Autodesk Inventor part; units mm, degrees
(part 10 of 13)
  spline S1362 degree 3 poles (18.9643, 15.7078) (18.9643, 15.461) (19.1644, 15.2608) (19.4112, 15.2608) knots 0 0 0 0 1 1 1 1
  line L4312 (18.9643, 15.7078) -> (18.9643, 15.461) construction
  line L4313 (18.9643, 15.461) -> (19.1644, 15.2608) construction
  line L4314 (19.1644, 15.2608) -> (19.4112, 15.2608) construction
  spline S1363 degree 3 poles (19.4112, 15.2608) (19.658, 15.2608) (19.8582, 15.461) (19.8582, 15.7078) knots 0 0 0 0 1 1 1 1
  line L4315 (19.4112, 15.2608) -> (19.658, 15.2608) construction
  line L4316 (19.658, 15.2608) -> (19.8582, 15.461) construction
  line L4317 (19.8582, 15.461) -> (19.8582, 15.7078) construction
  spline S1364 degree 3 poles (19.8582, 18.2619) (19.8582, 18.5087) (19.658, 18.7088) (19.4112, 18.7088) knots 0 0 0 0 1 1 1 1
  line L4318 (19.8582, 18.2619) -> (19.8582, 18.5087) construction
  line L4319 (19.8582, 18.5087) -> (19.658, 18.7088) construction
  line L4320 (19.658, 18.7088) -> (19.4112, 18.7088) construction
  spline S1365 degree 3 poles (19.4112, 18.7088) (19.1644, 18.7088) (18.9643, 18.5087) (18.9643, 18.2619) knots 0 0 0 0 1 1 1 1
  line L4321 (19.4112, 18.7088) -> (19.1644, 18.7088) construction
  line L4322 (19.1644, 18.7088) -> (18.9643, 18.5087) construction
  line L4323 (18.9643, 18.5087) -> (18.9643, 18.2619) construction
  spline S1366 degree 3 poles (18.9643, 18.2619) (18.9643, 18.0151) (19.1644, 17.8149) (19.4112, 17.8149) knots 0 0 0 0 1 1 1 1
  line L4324 (18.9643, 18.2619) -> (18.9643, 18.0151) construction
  line L4325 (18.9643, 18.0151) -> (19.1644, 17.8149) construction
  line L4326 (19.1644, 17.8149) -> (19.4112, 17.8149) construction
  spline S1367 degree 3 poles (19.4112, 17.8149) (19.658, 17.8149) (19.8582, 18.0151) (19.8582, 18.2619) knots 0 0 0 0 1 1 1 1
  line L4327 (19.4112, 17.8149) -> (19.658, 17.8149) construction
  line L4328 (19.658, 17.8149) -> (19.8582, 18.0151) construction
  line L4329 (19.8582, 18.0151) -> (19.8582, 18.2619) construction
  spline S1368 degree 3 poles (19.8582, 20.816) (19.8582, 21.0628) (19.658, 21.2629) (19.4112, 21.2629) knots 0 0 0 0 1 1 1 1
  line L4330 (19.8582, 20.816) -> (19.8582, 21.0628) construction
  line L4331 (19.8582, 21.0628) -> (19.658, 21.2629) construction
  line L4332 (19.658, 21.2629) -> (19.4112, 21.2629) construction
  spline S1369 degree 3 poles (19.4112, 21.2629) (19.1644, 21.2629) (18.9643, 21.0628) (18.9643, 20.816) knots 0 0 0 0 1 1 1 1
  line L4333 (19.4112, 21.2629) -> (19.1644, 21.2629) construction
  line L4334 (19.1644, 21.2629) -> (18.9643, 21.0628) construction
  line L4335 (18.9643, 21.0628) -> (18.9643, 20.816) construction
  spline S1370 degree 3 poles (18.9643, 20.816) (18.9643, 20.5692) (19.1644, 20.369) (19.4112, 20.369) knots 0 0 0 0 1 1 1 1
  line L4336 (18.9643, 20.816) -> (18.9643, 20.5692) construction
  line L4337 (18.9643, 20.5692) -> (19.1644, 20.369) construction
  line L4338 (19.1644, 20.369) -> (19.4112, 20.369) construction
  spline S1371 degree 3 poles (19.4112, 20.369) (19.658, 20.369) (19.8582, 20.5692) (19.8582, 20.816) knots 0 0 0 0 1 1 1 1
  line L4339 (19.4112, 20.369) -> (19.658, 20.369) construction
  line L4340 (19.658, 20.369) -> (19.8582, 20.5692) construction
  line L4341 (19.8582, 20.5692) -> (19.8582, 20.816) construction
  spline S1372 degree 3 poles (9.6418, 33.5866) (9.6418, 33.8334) (9.4415, 34.0334) (9.1948, 34.0334) knots 0 0 0 0 1 1 1 1
  line L4342 (9.6418, 33.5866) -> (9.6418, 33.8334) construction
  line L4343 (9.6418, 33.8334) -> (9.4415, 34.0334) construction
  line L4344 (9.4415, 34.0334) -> (9.1948, 34.0334) construction
  spline S1373 degree 3 poles (9.1948, 34.0334) (8.948, 34.0334) (8.7479, 33.8334) (8.7479, 33.5866) knots 0 0 0 0 1 1 1 1
  line L4345 (9.1948, 34.0334) -> (8.948, 34.0334) construction
  line L4346 (8.948, 34.0334) -> (8.7479, 33.8334) construction
  line L4347 (8.7479, 33.8334) -> (8.7479, 33.5866) construction
  spline S1374 degree 3 poles (8.7479, 33.5866) (8.7479, 33.3398) (8.948, 33.1395) (9.1948, 33.1395) knots 0 0 0 0 1 1 1 1
  line L4348 (8.7479, 33.5866) -> (8.7479, 33.3398) construction
  line L4349 (8.7479, 33.3398) -> (8.948, 33.1395) construction
  line L4350 (8.948, 33.1395) -> (9.1948, 33.1395) construction
  spline S1375 degree 3 poles (9.1948, 33.1395) (9.4415, 33.1395) (9.6418, 33.3398) (9.6418, 33.5866) knots 0 0 0 0 1 1 1 1
  line L4351 (9.1948, 33.1395) -> (9.4415, 33.1395) construction
  line L4352 (9.4415, 33.1395) -> (9.6418, 33.3398) construction
  line L4353 (9.6418, 33.3398) -> (9.6418, 33.5866) construction
  spline S1376 degree 3 poles (12.1959, 33.5866) (12.1959, 33.8334) (11.9957, 34.0334) (11.7489, 34.0334) knots 0 0 0 0 1 1 1 1
  line L4354 (12.1959, 33.5866) -> (12.1959, 33.8334) construction
  line L4355 (12.1959, 33.8334) -> (11.9957, 34.0334) construction
  line L4356 (11.9957, 34.0334) -> (11.7489, 34.0334) construction
  spline S1377 degree 3 poles (11.7489, 34.0334) (11.5021, 34.0334) (11.302, 33.8334) (11.302, 33.5866) knots 0 0 0 0 1 1 1 1
  line L4357 (11.7489, 34.0334) -> (11.5021, 34.0334) construction
  line L4358 (11.5021, 34.0334) -> (11.302, 33.8334) construction
  line L4359 (11.302, 33.8334) -> (11.302, 33.5866) construction
  spline S1378 degree 3 poles (11.302, 33.5866) (11.302, 33.3398) (11.5021, 33.1395) (11.7489, 33.1395) knots 0 0 0 0 1 1 1 1
  line L4360 (11.302, 33.5866) -> (11.302, 33.3398) construction
  line L4361 (11.302, 33.3398) -> (11.5021, 33.1395) construction
  line L4362 (11.5021, 33.1395) -> (11.7489, 33.1395) construction
  spline S1379 degree 3 poles (11.7489, 33.1395) (11.9957, 33.1395) (12.1959, 33.3398) (12.1959, 33.5866) knots 0 0 0 0 1 1 1 1
  line L4363 (11.7489, 33.1395) -> (11.9957, 33.1395) construction
  line L4364 (11.9957, 33.1395) -> (12.1959, 33.3398) construction
  line L4365 (12.1959, 33.3398) -> (12.1959, 33.5866) construction
  spline S1380 degree 3 poles (14.75, 33.5866) (14.75, 33.8334) (14.5498, 34.0334) (14.303, 34.0334) knots 0 0 0 0 1 1 1 1
  line L4366 (14.75, 33.5866) -> (14.75, 33.8334) construction
  line L4367 (14.75, 33.8334) -> (14.5498, 34.0334) construction
  line L4368 (14.5498, 34.0334) -> (14.303, 34.0334) construction
  spline S1381 degree 3 poles (14.303, 34.0334) (14.0562, 34.0334) (13.8561, 33.8334) (13.8561, 33.5866) knots 0 0 0 0 1 1 1 1
  line L4369 (14.303, 34.0334) -> (14.0562, 34.0334) construction
  line L4370 (14.0562, 34.0334) -> (13.8561, 33.8334) construction
  line L4371 (13.8561, 33.8334) -> (13.8561, 33.5866) construction
  spline S1382 degree 3 poles (13.8561, 33.5866) (13.8561, 33.3398) (14.0562, 33.1395) (14.303, 33.1395) knots 0 0 0 0 1 1 1 1
  line L4372 (13.8561, 33.5866) -> (13.8561, 33.3398) construction
  line L4373 (13.8561, 33.3398) -> (14.0562, 33.1395) construction
  line L4374 (14.0562, 33.1395) -> (14.303, 33.1395) construction
  spline S1383 degree 3 poles (14.303, 33.1395) (14.5498, 33.1395) (14.75, 33.3398) (14.75, 33.5866) knots 0 0 0 0 1 1 1 1
  line L4375 (14.303, 33.1395) -> (14.5498, 33.1395) construction
  line L4376 (14.5498, 33.1395) -> (14.75, 33.3398) construction
  line L4377 (14.75, 33.3398) -> (14.75, 33.5866) construction
  spline S1384 degree 3 poles (17.3041, 23.3701) (17.3041, 23.6169) (17.1039, 23.817) (16.8571, 23.817) knots 0 0 0 0 1 1 1 1
  line L4378 (17.3041, 23.3701) -> (17.3041, 23.6169) construction
  line L4379 (17.3041, 23.6169) -> (17.1039, 23.817) construction
  line L4380 (17.1039, 23.817) -> (16.8571, 23.817) construction
  spline S1385 degree 3 poles (16.8571, 23.817) (16.6103, 23.817) (16.4102, 23.6169) (16.4102, 23.3701) knots 0 0 0 0 1 1 1 1
  line L4381 (16.8571, 23.817) -> (16.6103, 23.817) construction
  line L4382 (16.6103, 23.817) -> (16.4102, 23.6169) construction
  line L4383 (16.4102, 23.6169) -> (16.4102, 23.3701) construction
  spline S1386 degree 3 poles (16.4102, 23.3701) (16.4102, 23.1233) (16.6103, 22.9231) (16.8571, 22.9231) knots 0 0 0 0 1 1 1 1
  line L4384 (16.4102, 23.3701) -> (16.4102, 23.1233) construction
  line L4385 (16.4102, 23.1233) -> (16.6103, 22.9231) construction
  line L4386 (16.6103, 22.9231) -> (16.8571, 22.9231) construction
  spline S1387 degree 3 poles (16.8571, 22.9231) (17.1039, 22.9231) (17.3041, 23.1233) (17.3041, 23.3701) knots 0 0 0 0 1 1 1 1
  line L4387 (16.8571, 22.9231) -> (17.1039, 22.9231) construction
  line L4388 (17.1039, 22.9231) -> (17.3041, 23.1233) construction
  line L4389 (17.3041, 23.1233) -> (17.3041, 23.3701) construction
  spline S1388 degree 3 poles (22.7955, 22.2718) (22.7955, 22.5186) (22.5952, 22.7188) (22.3485, 22.7188) knots 0 0 0 0 1 1 1 1
  line L4390 (22.7955, 22.2718) -> (22.7955, 22.5186) construction
  line L4391 (22.7955, 22.5186) -> (22.5952, 22.7188) construction
  line L4392 (22.5952, 22.7188) -> (22.3485, 22.7188) construction
  spline S1389 degree 3 poles (22.3485, 22.7188) (22.1017, 22.7188) (21.9014, 22.5186) (21.9014, 22.2718) knots 0 0 0 0 1 1 1 1
  line L4393 (22.3485, 22.7188) -> (22.1017, 22.7188) construction
  line L4394 (22.1017, 22.7188) -> (21.9014, 22.5186) construction
  line L4395 (21.9014, 22.5186) -> (21.9014, 22.2718) construction
  spline S1390 degree 3 poles (21.9014, 22.2718) (21.9014, 22.025) (22.1017, 21.8248) (22.3485, 21.8248) knots 0 0 0 0 1 1 1 1
  line L4396 (21.9014, 22.2718) -> (21.9014, 22.025) construction
  line L4397 (21.9014, 22.025) -> (22.1017, 21.8248) construction
  line L4398 (22.1017, 21.8248) -> (22.3485, 21.8248) construction
  spline S1391 degree 3 poles (22.3485, 21.8248) (22.5952, 21.8248) (22.7955, 22.025) (22.7955, 22.2718) knots 0 0 0 0 1 1 1 1
  line L4399 (22.3485, 21.8248) -> (22.5952, 21.8248) construction
  line L4400 (22.5952, 21.8248) -> (22.7955, 22.025) construction
  line L4401 (22.7955, 22.025) -> (22.7955, 22.2718) construction
  spline S1392 degree 3 poles (25.3496, 22.2718) (25.3496, 22.5186) (25.1494, 22.7188) (24.9026, 22.7188) knots 0 0 0 0 1 1 1 1
  line L4402 (25.3496, 22.2718) -> (25.3496, 22.5186) construction
  line L4403 (25.3496, 22.5186) -> (25.1494, 22.7188) construction
  line L4404 (25.1494, 22.7188) -> (24.9026, 22.7188) construction
  spline S1393 degree 3 poles (24.9026, 22.7188) (24.6558, 22.7188) (24.4555, 22.5186) (24.4555, 22.2718) knots 0 0 0 0 1 1 1 1
  line L4405 (24.9026, 22.7188) -> (24.6558, 22.7188) construction
  line L4406 (24.6558, 22.7188) -> (24.4555, 22.5186) construction
  line L4407 (24.4555, 22.5186) -> (24.4555, 22.2718) construction
  spline S1394 degree 3 poles (24.4555, 22.2718) (24.4555, 22.025) (24.6558, 21.8248) (24.9026, 21.8248) knots 0 0 0 0 1 1 1 1
  line L4408 (24.4555, 22.2718) -> (24.4555, 22.025) construction
  line L4409 (24.4555, 22.025) -> (24.6558, 21.8248) construction
  line L4410 (24.6558, 21.8248) -> (24.9026, 21.8248) construction
  spline S1395 degree 3 poles (24.9026, 21.8248) (25.1494, 21.8248) (25.3496, 22.025) (25.3496, 22.2718) knots 0 0 0 0 1 1 1 1
  line L4411 (24.9026, 21.8248) -> (25.1494, 21.8248) construction
  line L4412 (25.1494, 21.8248) -> (25.3496, 22.025) construction
  line L4413 (25.3496, 22.025) -> (25.3496, 22.2718) construction
  spline S1396 degree 3 poles (22.7955, 24.8259) (22.7955, 25.0727) (22.5952, 25.2729) (22.3485, 25.2729) knots 0 0 0 0 1 1 1 1
  line L4414 (22.7955, 24.8259) -> (22.7955, 25.0727) construction
  line L4415 (22.7955, 25.0727) -> (22.5952, 25.2729) construction
  line L4416 (22.5952, 25.2729) -> (22.3485, 25.2729) construction
  spline S1397 degree 3 poles (22.3485, 25.2729) (22.1017, 25.2729) (21.9014, 25.0727) (21.9014, 24.8259) knots 0 0 0 0 1 1 1 1
  line L4417 (22.3485, 25.2729) -> (22.1017, 25.2729) construction
  line L4418 (22.1017, 25.2729) -> (21.9014, 25.0727) construction
  line L4419 (21.9014, 25.0727) -> (21.9014, 24.8259) construction
  spline S1398 degree 3 poles (21.9014, 24.8259) (21.9014, 24.5792) (22.1017, 24.3789) (22.3485, 24.3789) knots 0 0 0 0 1 1 1 1
  line L4420 (21.9014, 24.8259) -> (21.9014, 24.5792) construction
  line L4421 (21.9014, 24.5792) -> (22.1017, 24.3789) construction
  line L4422 (22.1017, 24.3789) -> (22.3485, 24.3789) construction
  spline S1399 degree 3 poles (22.3485, 24.3789) (22.5952, 24.3789) (22.7955, 24.5792) (22.7955, 24.8259) knots 0 0 0 0 1 1 1 1
  line L4423 (22.3485, 24.3789) -> (22.5952, 24.3789) construction
  line L4424 (22.5952, 24.3789) -> (22.7955, 24.5792) construction
  line L4425 (22.7955, 24.5792) -> (22.7955, 24.8259) construction
  spline S1400 degree 3 poles (25.3496, 24.8259) (25.3496, 25.0727) (25.1494, 25.2729) (24.9026, 25.2729) knots 0 0 0 0 1 1 1 1
  line L4426 (25.3496, 24.8259) -> (25.3496, 25.0727) construction
  line L4427 (25.3496, 25.0727) -> (25.1494, 25.2729) construction
  line L4428 (25.1494, 25.2729) -> (24.9026, 25.2729) construction
  spline S1401 degree 3 poles (24.9026, 25.2729) (24.6558, 25.2729) (24.4555, 25.0727) (24.4555, 24.8259) knots 0 0 0 0 1 1 1 1
  line L4429 (24.9026, 25.2729) -> (24.6558, 25.2729) construction
  line L4430 (24.6558, 25.2729) -> (24.4555, 25.0727) construction
  line L4431 (24.4555, 25.0727) -> (24.4555, 24.8259) construction
  spline S1402 degree 3 poles (24.4555, 24.8259) (24.4555, 24.5792) (24.6558, 24.3789) (24.9026, 24.3789) knots 0 0 0 0 1 1 1 1
  line L4432 (24.4555, 24.8259) -> (24.4555, 24.5792) construction
  line L4433 (24.4555, 24.5792) -> (24.6558, 24.3789) construction
  line L4434 (24.6558, 24.3789) -> (24.9026, 24.3789) construction
  spline S1403 degree 3 poles (24.9026, 24.3789) (25.1494, 24.3789) (25.3496, 24.5792) (25.3496, 24.8259) knots 0 0 0 0 1 1 1 1
  line L4435 (24.9026, 24.3789) -> (25.1494, 24.3789) construction
  line L4436 (25.1494, 24.3789) -> (25.3496, 24.5792) construction
  line L4437 (25.3496, 24.5792) -> (25.3496, 24.8259) construction
  spline S1404 degree 3 poles (19.8582, 23.3701) (19.8582, 23.6169) (19.658, 23.817) (19.4112, 23.817) knots 0 0 0 0 1 1 1 1
  line L4438 (19.8582, 23.3701) -> (19.8582, 23.6169) construction
  line L4439 (19.8582, 23.6169) -> (19.658, 23.817) construction
  line L4440 (19.658, 23.817) -> (19.4112, 23.817) construction
  spline S1405 degree 3 poles (19.4112, 23.817) (19.1644, 23.817) (18.9643, 23.6169) (18.9643, 23.3701) knots 0 0 0 0 1 1 1 1
  line L4441 (19.4112, 23.817) -> (19.1644, 23.817) construction
  line L4442 (19.1644, 23.817) -> (18.9643, 23.6169) construction
  line L4443 (18.9643, 23.6169) -> (18.9643, 23.3701) construction
  spline S1406 degree 3 poles (18.9643, 23.3701) (18.9643, 23.1233) (19.1644, 22.9231) (19.4112, 22.9231) knots 0 0 0 0 1 1 1 1
  line L4444 (18.9643, 23.3701) -> (18.9643, 23.1233) construction
  line L4445 (18.9643, 23.1233) -> (19.1644, 22.9231) construction
  line L4446 (19.1644, 22.9231) -> (19.4112, 22.9231) construction
  spline S1407 degree 3 poles (19.4112, 22.9231) (19.658, 22.9231) (19.8582, 23.1233) (19.8582, 23.3701) knots 0 0 0 0 1 1 1 1
  line L4447 (19.4112, 22.9231) -> (19.658, 22.9231) construction
  line L4448 (19.658, 22.9231) -> (19.8582, 23.1233) construction
  line L4449 (19.8582, 23.1233) -> (19.8582, 23.3701) construction
  spline S1408 degree 3 poles (19.8582, 25.9242) (19.8582, 26.171) (19.658, 26.3711) (19.4112, 26.3711) knots 0 0 0 0 1 1 1 1
  line L4450 (19.8582, 25.9242) -> (19.8582, 26.171) construction
  line L4451 (19.8582, 26.171) -> (19.658, 26.3711) construction
  line L4452 (19.658, 26.3711) -> (19.4112, 26.3711) construction
  spline S1409 degree 3 poles (19.4112, 26.3711) (19.1644, 26.3711) (18.9643, 26.171) (18.9643, 25.9242) knots 0 0 0 0 1 1 1 1
  line L4453 (19.4112, 26.3711) -> (19.1644, 26.3711) construction
  line L4454 (19.1644, 26.3711) -> (18.9643, 26.171) construction
  line L4455 (18.9643, 26.171) -> (18.9643, 25.9242) construction
  spline S1410 degree 3 poles (18.9643, 25.9242) (18.9643, 25.6775) (19.1644, 25.4772) (19.4112, 25.4772) knots 0 0 0 0 1 1 1 1
  line L4456 (18.9643, 25.9242) -> (18.9643, 25.6775) construction
  line L4457 (18.9643, 25.6775) -> (19.1644, 25.4772) construction
  line L4458 (19.1644, 25.4772) -> (19.4112, 25.4772) construction
  spline S1411 degree 3 poles (19.4112, 25.4772) (19.658, 25.4772) (19.8582, 25.6775) (19.8582, 25.9242) knots 0 0 0 0 1 1 1 1
  line L4459 (19.4112, 25.4772) -> (19.658, 25.4772) construction
  line L4460 (19.658, 25.4772) -> (19.8582, 25.6775) construction
  line L4461 (19.8582, 25.6775) -> (19.8582, 25.9242) construction
  spline S1412 degree 3 poles (19.8582, 28.4784) (19.8582, 28.7251) (19.658, 28.9252) (19.4112, 28.9252) knots 0 0 0 0 1 1 1 1
  line L4462 (19.8582, 28.4784) -> (19.8582, 28.7251) construction
  line L4463 (19.8582, 28.7251) -> (19.658, 28.9252) construction
  line L4464 (19.658, 28.9252) -> (19.4112, 28.9252) construction
  spline S1413 degree 3 poles (19.4112, 28.9252) (19.1644, 28.9252) (18.9643, 28.7251) (18.9643, 28.4784) knots 0 0 0 0 1 1 1 1
  line L4465 (19.4112, 28.9252) -> (19.1644, 28.9252) construction
  line L4466 (19.1644, 28.9252) -> (18.9643, 28.7251) construction
  line L4467 (18.9643, 28.7251) -> (18.9643, 28.4784) construction
  spline S1414 degree 3 poles (18.9643, 28.4784) (18.9643, 28.2316) (19.1644, 28.0313) (19.4112, 28.0313) knots 0 0 0 0 1 1 1 1
  line L4468 (18.9643, 28.4784) -> (18.9643, 28.2316) construction
  line L4469 (18.9643, 28.2316) -> (19.1644, 28.0313) construction
  line L4470 (19.1644, 28.0313) -> (19.4112, 28.0313) construction
  spline S1415 degree 3 poles (19.4112, 28.0313) (19.658, 28.0313) (19.8582, 28.2316) (19.8582, 28.4784) knots 0 0 0 0 1 1 1 1
  line L4471 (19.4112, 28.0313) -> (19.658, 28.0313) construction
  line L4472 (19.658, 28.0313) -> (19.8582, 28.2316) construction
  line L4473 (19.8582, 28.2316) -> (19.8582, 28.4784) construction
  spline S1416 degree 3 poles (19.8582, 31.0325) (19.8582, 31.2793) (19.658, 31.4793) (19.4112, 31.4793) knots 0 0 0 0 1 1 1 1
  line L4474 (19.8582, 31.0325) -> (19.8582, 31.2793) construction
  line L4475 (19.8582, 31.2793) -> (19.658, 31.4793) construction
  line L4476 (19.658, 31.4793) -> (19.4112, 31.4793) construction
  spline S1417 degree 3 poles (19.4112, 31.4793) (19.1644, 31.4793) (18.9643, 31.2793) (18.9643, 31.0325) knots 0 0 0 0 1 1 1 1
  line L4477 (19.4112, 31.4793) -> (19.1644, 31.4793) construction
  line L4478 (19.1644, 31.4793) -> (18.9643, 31.2793) construction
  line L4479 (18.9643, 31.2793) -> (18.9643, 31.0325) construction
  spline S1418 degree 3 poles (18.9643, 31.0325) (18.9643, 30.7857) (19.1644, 30.5854) (19.4112, 30.5854) knots 0 0 0 0 1 1 1 1
  line L4480 (18.9643, 31.0325) -> (18.9643, 30.7857) construction
  line L4481 (18.9643, 30.7857) -> (19.1644, 30.5854) construction
  line L4482 (19.1644, 30.5854) -> (19.4112, 30.5854) construction
  spline S1419 degree 3 poles (19.4112, 30.5854) (19.658, 30.5854) (19.8582, 30.7857) (19.8582, 31.0325) knots 0 0 0 0 1 1 1 1
  line L4483 (19.4112, 30.5854) -> (19.658, 30.5854) construction
  line L4484 (19.658, 30.5854) -> (19.8582, 30.7857) construction
  line L4485 (19.8582, 30.7857) -> (19.8582, 31.0325) construction
  spline S1420 degree 3 poles (17.3041, 25.9242) (17.3041, 26.171) (17.1039, 26.3711) (16.8571, 26.3711) knots 0 0 0 0 1 1 1 1
  line L4486 (17.3041, 25.9242) -> (17.3041, 26.171) construction
  line L4487 (17.3041, 26.171) -> (17.1039, 26.3711) construction
  line L4488 (17.1039, 26.3711) -> (16.8571, 26.3711) construction
  spline S1421 degree 3 poles (16.8571, 26.3711) (16.6103, 26.3711) (16.4102, 26.171) (16.4102, 25.9242) knots 0 0 0 0 1 1 1 1
  line L4489 (16.8571, 26.3711) -> (16.6103, 26.3711) construction
  line L4490 (16.6103, 26.3711) -> (16.4102, 26.171) construction
  line L4491 (16.4102, 26.171) -> (16.4102, 25.9242) construction
  spline S1422 degree 3 poles (16.4102, 25.9242) (16.4102, 25.6775) (16.6103, 25.4772) (16.8571, 25.4772) knots 0 0 0 0 1 1 1 1
  line L4492 (16.4102, 25.9242) -> (16.4102, 25.6775) construction
  line L4493 (16.4102, 25.6775) -> (16.6103, 25.4772) construction
  line L4494 (16.6103, 25.4772) -> (16.8571, 25.4772) construction
  spline S1423 degree 3 poles (16.8571, 25.4772) (17.1039, 25.4772) (17.3041, 25.6775) (17.3041, 25.9242) knots 0 0 0 0 1 1 1 1
  line L4495 (16.8571, 25.4772) -> (17.1039, 25.4772) construction
  line L4496 (17.1039, 25.4772) -> (17.3041, 25.6775) construction
  line L4497 (17.3041, 25.6775) -> (17.3041, 25.9242) construction
  spline S1424 degree 3 poles (17.3041, 28.4784) (17.3041, 28.7251) (17.1039, 28.9252) (16.8571, 28.9252) knots 0 0 0 0 1 1 1 1
  line L4498 (17.3041, 28.4784) -> (17.3041, 28.7251) construction
  line L4499 (17.3041, 28.7251) -> (17.1039, 28.9252) construction
  line L4500 (17.1039, 28.9252) -> (16.8571, 28.9252) construction
  spline S1425 degree 3 poles (16.8571, 28.9252) (16.6103, 28.9252) (16.4102, 28.7251) (16.4102, 28.4784) knots 0 0 0 0 1 1 1 1
  line L4501 (16.8571, 28.9252) -> (16.6103, 28.9252) construction
  line L4502 (16.6103, 28.9252) -> (16.4102, 28.7251) construction
  line L4503 (16.4102, 28.7251) -> (16.4102, 28.4784) construction
  spline S1426 degree 3 poles (16.4102, 28.4784) (16.4102, 28.2316) (16.6103, 28.0313) (16.8571, 28.0313) knots 0 0 0 0 1 1 1 1
  line L4504 (16.4102, 28.4784) -> (16.4102, 28.2316) construction
  line L4505 (16.4102, 28.2316) -> (16.6103, 28.0313) construction
  line L4506 (16.6103, 28.0313) -> (16.8571, 28.0313) construction
  spline S1427 degree 3 poles (16.8571, 28.0313) (17.1039, 28.0313) (17.3041, 28.2316) (17.3041, 28.4784) knots 0 0 0 0 1 1 1 1
  line L4507 (16.8571, 28.0313) -> (17.1039, 28.0313) construction
  line L4508 (17.1039, 28.0313) -> (17.3041, 28.2316) construction
  line L4509 (17.3041, 28.2316) -> (17.3041, 28.4784) construction
  spline S1428 degree 3 poles (17.3041, 31.0325) (17.3041, 31.2793) (17.1039, 31.4793) (16.8571, 31.4793) knots 0 0 0 0 1 1 1 1
  line L4510 (17.3041, 31.0325) -> (17.3041, 31.2793) construction
  line L4511 (17.3041, 31.2793) -> (17.1039, 31.4793) construction
  line L4512 (17.1039, 31.4793) -> (16.8571, 31.4793) construction
  spline S1429 degree 3 poles (16.8571, 31.4793) (16.6103, 31.4793) (16.4102, 31.2793) (16.4102, 31.0325) knots 0 0 0 0 1 1 1 1
  line L4513 (16.8571, 31.4793) -> (16.6103, 31.4793) construction
  line L4514 (16.6103, 31.4793) -> (16.4102, 31.2793) construction
  line L4515 (16.4102, 31.2793) -> (16.4102, 31.0325) construction
  spline S1430 degree 3 poles (16.4102, 31.0325) (16.4102, 30.7857) (16.6103, 30.5854) (16.8571, 30.5854) knots 0 0 0 0 1 1 1 1
  line L4516 (16.4102, 31.0325) -> (16.4102, 30.7857) construction
  line L4517 (16.4102, 30.7857) -> (16.6103, 30.5854) construction
  line L4518 (16.6103, 30.5854) -> (16.8571, 30.5854) construction
  spline S1431 degree 3 poles (16.8571, 30.5854) (17.1039, 30.5854) (17.3041, 30.7857) (17.3041, 31.0325) knots 0 0 0 0 1 1 1 1
  line L4519 (16.8571, 30.5854) -> (17.1039, 30.5854) construction
  line L4520 (17.1039, 30.5854) -> (17.3041, 30.7857) construction
  line L4521 (17.3041, 30.7857) -> (17.3041, 31.0325) construction
  spline S1432 degree 3 poles (37.737, 33.5866) (37.737, 33.8334) (37.5369, 34.0334) (37.29, 34.0334) knots 0 0 0 0 1 1 1 1
  line L4522 (37.737, 33.5866) -> (37.737, 33.8334) construction
  line L4523 (37.737, 33.8334) -> (37.5369, 34.0334) construction
  line L4524 (37.5369, 34.0334) -> (37.29, 34.0334) construction
  spline S1433 degree 3 poles (37.29, 34.0334) (37.0431, 34.0334) (36.843, 33.8334) (36.843, 33.5866) knots 0 0 0 0 1 1 1 1
  line L4525 (37.29, 34.0334) -> (37.0431, 34.0334) construction
  line L4526 (37.0431, 34.0334) -> (36.843, 33.8334) construction
  line L4527 (36.843, 33.8334) -> (36.843, 33.5866) construction
  spline S1434 degree 3 poles (36.843, 33.5866) (36.843, 33.3398) (37.0431, 33.1395) (37.29, 33.1395) knots 0 0 0 0 1 1 1 1
  line L4528 (36.843, 33.5866) -> (36.843, 33.3398) construction
  line L4529 (36.843, 33.3398) -> (37.0431, 33.1395) construction
  line L4530 (37.0431, 33.1395) -> (37.29, 33.1395) construction
  spline S1435 degree 3 poles (37.29, 33.1395) (37.5369, 33.1395) (37.737, 33.3398) (37.737, 33.5866) knots 0 0 0 0 1 1 1 1
  line L4531 (37.29, 33.1395) -> (37.5369, 33.1395) construction
  line L4532 (37.5369, 33.1395) -> (37.737, 33.3398) construction
  line L4533 (37.737, 33.3398) -> (37.737, 33.5866) construction
  spline S1436 degree 3 poles (40.2911, 33.5866) (40.2911, 33.8334) (40.091, 34.0334) (39.8441, 34.0334) knots 0 0 0 0 1 1 1 1
  line L4534 (40.2911, 33.5866) -> (40.2911, 33.8334) construction
  line L4535 (40.2911, 33.8334) -> (40.091, 34.0334) construction
  line L4536 (40.091, 34.0334) -> (39.8441, 34.0334) construction
  spline S1437 degree 3 poles (39.8441, 34.0334) (39.5972, 34.0334) (39.3971, 33.8334) (39.3971, 33.5866) knots 0 0 0 0 1 1 1 1
  line L4537 (39.8441, 34.0334) -> (39.5972, 34.0334) construction
  line L4538 (39.5972, 34.0334) -> (39.3971, 33.8334) construction
  line L4539 (39.3971, 33.8334) -> (39.3971, 33.5866) construction
  spline S1438 degree 3 poles (39.3971, 33.5866) (39.3971, 33.3398) (39.5972, 33.1395) (39.8441, 33.1395) knots 0 0 0 0 1 1 1 1
  line L4540 (39.3971, 33.5866) -> (39.3971, 33.3398) construction
  line L4541 (39.3971, 33.3398) -> (39.5972, 33.1395) construction
  line L4542 (39.5972, 33.1395) -> (39.8441, 33.1395) construction
  spline S1439 degree 3 poles (39.8441, 33.1395) (40.091, 33.1395) (40.2911, 33.3398) (40.2911, 33.5866) knots 0 0 0 0 1 1 1 1
  line L4543 (39.8441, 33.1395) -> (40.091, 33.1395) construction
  line L4544 (40.091, 33.1395) -> (40.2911, 33.3398) construction
  line L4545 (40.2911, 33.3398) -> (40.2911, 33.5866) construction
  spline S1440 degree 3 poles (42.8452, 33.5866) (42.8452, 33.8334) (42.6451, 34.0334) (42.3982, 34.0334) knots 0 0 0 0 1 1 1 1
  line L4546 (42.8452, 33.5866) -> (42.8452, 33.8334) construction
  line L4547 (42.8452, 33.8334) -> (42.6451, 34.0334) construction
  line L4548 (42.6451, 34.0334) -> (42.3982, 34.0334) construction
  spline S1441 degree 3 poles (42.3982, 34.0334) (42.1513, 34.0334) (41.9512, 33.8334) (41.9512, 33.5866) knots 0 0 0 0 1 1 1 1
  line L4549 (42.3982, 34.0334) -> (42.1513, 34.0334) construction
  line L4550 (42.1513, 34.0334) -> (41.9512, 33.8334) construction
  line L4551 (41.9512, 33.8334) -> (41.9512, 33.5866) construction
  spline S1442 degree 3 poles (41.9512, 33.5866) (41.9512, 33.3398) (42.1513, 33.1395) (42.3982, 33.1395) knots 0 0 0 0 1 1 1 1
  line L4552 (41.9512, 33.5866) -> (41.9512, 33.3398) construction
  line L4553 (41.9512, 33.3398) -> (42.1513, 33.1395) construction
  line L4554 (42.1513, 33.1395) -> (42.3982, 33.1395) construction
  spline S1443 degree 3 poles (42.3982, 33.1395) (42.6451, 33.1395) (42.8452, 33.3398) (42.8452, 33.5866) knots 0 0 0 0 1 1 1 1
  line L4555 (42.3982, 33.1395) -> (42.6451, 33.1395) construction
  line L4556 (42.6451, 33.1395) -> (42.8452, 33.3398) construction
  line L4557 (42.8452, 33.3398) -> (42.8452, 33.5866) construction
  spline S1444 degree 3 poles (45.3993, 33.5866) (45.3993, 33.8334) (45.1992, 34.0334) (44.9523, 34.0334) knots 0 0 0 0 1 1 1 1
  line L4558 (45.3993, 33.5866) -> (45.3993, 33.8334) construction
  line L4559 (45.3993, 33.8334) -> (45.1992, 34.0334) construction
  line L4560 (45.1992, 34.0334) -> (44.9523, 34.0334) construction
  spline S1445 degree 3 poles (44.9523, 34.0334) (44.7054, 34.0334) (44.5054, 33.8334) (44.5054, 33.5866) knots 0 0 0 0 1 1 1 1
  line L4561 (44.9523, 34.0334) -> (44.7054, 34.0334) construction
  line L4562 (44.7054, 34.0334) -> (44.5054, 33.8334) construction
  line L4563 (44.5054, 33.8334) -> (44.5054, 33.5866) construction
  spline S1446 degree 3 poles (44.5054, 33.5866) (44.5054, 33.3398) (44.7054, 33.1395) (44.9523, 33.1395) knots 0 0 0 0 1 1 1 1
  line L4564 (44.5054, 33.5866) -> (44.5054, 33.3398) construction
  line L4565 (44.5054, 33.3398) -> (44.7054, 33.1395) construction
  line L4566 (44.7054, 33.1395) -> (44.9523, 33.1395) construction
  spline S1447 degree 3 poles (44.9523, 33.1395) (45.1992, 33.1395) (45.3993, 33.3398) (45.3993, 33.5866) knots 0 0 0 0 1 1 1 1
  line L4567 (44.9523, 33.1395) -> (45.1992, 33.1395) construction
  line L4568 (45.1992, 33.1395) -> (45.3993, 33.3398) construction
  line L4569 (45.3993, 33.3398) -> (45.3993, 33.5866) construction
  spline S1448 degree 3 poles (33.9058, 0.3832) (33.9058, 0.6299) (33.7056, 0.83) (33.4588, 0.83) knots 0 0 0 0 1 1 1 1
  line L4570 (33.9058, 0.3832) -> (33.9058, 0.6299) construction
  line L4571 (33.9058, 0.6299) -> (33.7056, 0.83) construction
  line L4572 (33.7056, 0.83) -> (33.4588, 0.83) construction
  spline S1449 degree 3 poles (33.4588, 0.83) (33.212, 0.83) (33.0119, 0.6299) (33.0119, 0.3832) knots 0 0 0 0 1 1 1 1
  line L4573 (33.4588, 0.83) -> (33.212, 0.83) construction
  line L4574 (33.212, 0.83) -> (33.0119, 0.6299) construction
  line L4575 (33.0119, 0.6299) -> (33.0119, 0.3832) construction
  spline S1450 degree 3 poles (33.0119, 0.3832) (33.0119, 0.1364) (33.212, -0.0639) (33.4588, -0.0639) knots 0 0 0 0 1 1 1 1
  line L4576 (33.0119, 0.3832) -> (33.0119, 0.1364) construction
  line L4577 (33.0119, 0.1364) -> (33.212, -0.0639) construction
  line L4578 (33.212, -0.0639) -> (33.4588, -0.0639) construction
  spline S1451 degree 3 poles (33.4588, -0.0639) (33.7056, -0.0639) (33.9058, 0.1364) (33.9058, 0.3832) knots 0 0 0 0 1 1 1 1
  line L4579 (33.4588, -0.0639) -> (33.7056, -0.0639) construction
  line L4580 (33.7056, -0.0639) -> (33.9058, 0.1364) construction
  line L4581 (33.9058, 0.1364) -> (33.9058, 0.3832) construction
  spline S1452 degree 3 poles (31.3517, 0.3832) (31.3517, 0.6299) (31.1515, 0.83) (30.9047, 0.83) knots 0 0 0 0 1 1 1 1
  line L4582 (31.3517, 0.3832) -> (31.3517, 0.6299) construction
  line L4583 (31.3517, 0.6299) -> (31.1515, 0.83) construction
  line L4584 (31.1515, 0.83) -> (30.9047, 0.83) construction
  spline S1453 degree 3 poles (30.9047, 0.83) (30.6579, 0.83) (30.4578, 0.6299) (30.4578, 0.3832) knots 0 0 0 0 1 1 1 1
  line L4585 (30.9047, 0.83) -> (30.6579, 0.83) construction
  line L4586 (30.6579, 0.83) -> (30.4578, 0.6299) construction
  line L4587 (30.4578, 0.6299) -> (30.4578, 0.3832) construction
  spline S1454 degree 3 poles (30.4578, 0.3832) (30.4578, 0.1364) (30.6579, -0.0639) (30.9047, -0.0639) knots 0 0 0 0 1 1 1 1
  line L4588 (30.4578, 0.3832) -> (30.4578, 0.1364) construction
  line L4589 (30.4578, 0.1364) -> (30.6579, -0.0639) construction
  line L4590 (30.6579, -0.0639) -> (30.9047, -0.0639) construction
  spline S1455 degree 3 poles (30.9047, -0.0639) (31.1515, -0.0639) (31.3517, 0.1364) (31.3517, 0.3832) knots 0 0 0 0 1 1 1 1
  line L4591 (30.9047, -0.0639) -> (31.1515, -0.0639) construction
  line L4592 (31.1515, -0.0639) -> (31.3517, 0.1364) construction
  line L4593 (31.3517, 0.1364) -> (31.3517, 0.3832) construction
  spline S1456 degree 3 poles (28.7976, 0.3832) (28.7976, 0.6299) (28.5974, 0.83) (28.3506, 0.83) knots 0 0 0 0 1 1 1 1
  line L4594 (28.7976, 0.3832) -> (28.7976, 0.6299) construction
  line L4595 (28.7976, 0.6299) -> (28.5974, 0.83) construction
  line L4596 (28.5974, 0.83) -> (28.3506, 0.83) construction
  spline S1457 degree 3 poles (28.3506, 0.83) (28.1038, 0.83) (27.9037, 0.6299) (27.9037, 0.3832) knots 0 0 0 0 1 1 1 1
  line L4597 (28.3506, 0.83) -> (28.1038, 0.83) construction
  line L4598 (28.1038, 0.83) -> (27.9037, 0.6299) construction
  line L4599 (27.9037, 0.6299) -> (27.9037, 0.3832) construction
  spline S1458 degree 3 poles (27.9037, 0.3832) (27.9037, 0.1364) (28.1038, -0.0639) (28.3506, -0.0639) knots 0 0 0 0 1 1 1 1
  line L4600 (27.9037, 0.3832) -> (27.9037, 0.1364) construction
  line L4601 (27.9037, 0.1364) -> (28.1038, -0.0639) construction
  line L4602 (28.1038, -0.0639) -> (28.3506, -0.0639) construction
  spline S1459 degree 3 poles (28.3506, -0.0639) (28.5974, -0.0639) (28.7976, 0.1364) (28.7976, 0.3832) knots 0 0 0 0 1 1 1 1
  line L4603 (28.3506, -0.0639) -> (28.5974, -0.0639) construction
  line L4604 (28.5974, -0.0639) -> (28.7976, 0.1364) construction
  line L4605 (28.7976, 0.1364) -> (28.7976, 0.3832) construction
  spline S1460 degree 3 poles (42.8452, 0.3832) (42.8452, 0.6299) (42.6451, 0.83) (42.3982, 0.83) knots 0 0 0 0 1 1 1 1
  line L4606 (42.8452, 0.3832) -> (42.8452, 0.6299) construction
  line L4607 (42.8452, 0.6299) -> (42.6451, 0.83) construction
  line L4608 (42.6451, 0.83) -> (42.3982, 0.83) construction
  spline S1461 degree 3 poles (42.3982, 0.83) (42.1513, 0.83) (41.9512, 0.6299) (41.9512, 0.3832) knots 0 0 0 0 1 1 1 1
  line L4609 (42.3982, 0.83) -> (42.1513, 0.83) construction
  line L4610 (42.1513, 0.83) -> (41.9512, 0.6299) construction
  line L4611 (41.9512, 0.6299) -> (41.9512, 0.3832) construction
  spline S1462 degree 3 poles (41.9512, 0.3832) (41.9512, 0.1364) (42.1513, -0.0639) (42.3982, -0.0639) knots 0 0 0 0 1 1 1 1
  line L4612 (41.9512, 0.3832) -> (41.9512, 0.1364) construction
  line L4613 (41.9512, 0.1364) -> (42.1513, -0.0639) construction
  line L4614 (42.1513, -0.0639) -> (42.3982, -0.0639) construction
  spline S1463 degree 3 poles (42.3982, -0.0639) (42.6451, -0.0639) (42.8452, 0.1364) (42.8452, 0.3832) knots 0 0 0 0 1 1 1 1
  line L4615 (42.3982, -0.0639) -> (42.6451, -0.0639) construction
  line L4616 (42.6451, -0.0639) -> (42.8452, 0.1364) construction
  line L4617 (42.8452, 0.1364) -> (42.8452, 0.3832) construction
  spline S1464 degree 3 poles (35.1829, 2.9373) (35.1829, 3.1841) (34.9826, 3.3841) (34.7358, 3.3841) knots 0 0 0 0 1 1 1 1
  line L4618 (35.1829, 2.9373) -> (35.1829, 3.1841) construction
  line L4619 (35.1829, 3.1841) -> (34.9826, 3.3841) construction
  line L4620 (34.9826, 3.3841) -> (34.7358, 3.3841) construction
  spline S1465 degree 3 poles (34.7358, 3.3841) (34.4891, 3.3841) (34.289, 3.1841) (34.289, 2.9373) knots 0 0 0 0 1 1 1 1
  line L4621 (34.7358, 3.3841) -> (34.4891, 3.3841) construction
  line L4622 (34.4891, 3.3841) -> (34.289, 3.1841) construction
  line L4623 (34.289, 3.1841) -> (34.289, 2.9373) construction
  spline S1466 degree 3 poles (34.289, 2.9373) (34.289, 2.6905) (34.4891, 2.4902) (34.7358, 2.4902) knots 0 0 0 0 1 1 1 1
  line L4624 (34.289, 2.9373) -> (34.289, 2.6905) construction
  line L4625 (34.289, 2.6905) -> (34.4891, 2.4902) construction
  line L4626 (34.4891, 2.4902) -> (34.7358, 2.4902) construction
  spline S1467 degree 3 poles (34.7358, 2.4902) (34.9826, 2.4902) (35.1829, 2.6905) (35.1829, 2.9373) knots 0 0 0 0 1 1 1 1
  line L4627 (34.7358, 2.4902) -> (34.9826, 2.4902) construction
  line L4628 (34.9826, 2.4902) -> (35.1829, 2.6905) construction
  line L4629 (35.1829, 2.6905) -> (35.1829, 2.9373) construction
  spline S1468 degree 3 poles (35.1829, 5.4914) (35.1829, 5.7382) (34.9826, 5.9382) (34.7358, 5.9382) knots 0 0 0 0 1 1 1 1
  line L4630 (35.1829, 5.4914) -> (35.1829, 5.7382) construction
  line L4631 (35.1829, 5.7382) -> (34.9826, 5.9382) construction
  line L4632 (34.9826, 5.9382) -> (34.7358, 5.9382) construction
  spline S1469 degree 3 poles (34.7358, 5.9382) (34.4891, 5.9382) (34.289, 5.7382) (34.289, 5.4914) knots 0 0 0 0 1 1 1 1
  line L4633 (34.7358, 5.9382) -> (34.4891, 5.9382) construction
  line L4634 (34.4891, 5.9382) -> (34.289, 5.7382) construction
  line L4635 (34.289, 5.7382) -> (34.289, 5.4914) construction
  spline S1470 degree 3 poles (34.289, 5.4914) (34.289, 5.2446) (34.4891, 5.0443) (34.7358, 5.0443) knots 0 0 0 0 1 1 1 1
  line L4636 (34.289, 5.4914) -> (34.289, 5.2446) construction
  line L4637 (34.289, 5.2446) -> (34.4891, 5.0443) construction
  line L4638 (34.4891, 5.0443) -> (34.7358, 5.0443) construction
  spline S1471 degree 3 poles (34.7358, 5.0443) (34.9826, 5.0443) (35.1829, 5.2446) (35.1829, 5.4914) knots 0 0 0 0 1 1 1 1
  line L4639 (34.7358, 5.0443) -> (34.9826, 5.0443) construction
  line L4640 (34.9826, 5.0443) -> (35.1829, 5.2446) construction
  line L4641 (35.1829, 5.2446) -> (35.1829, 5.4914) construction
  spline S1472 degree 3 poles (37.737, 5.4914) (37.737, 5.7382) (37.5369, 5.9382) (37.29, 5.9382) knots 0 0 0 0 1 1 1 1
  line L4642 (37.737, 5.4914) -> (37.737, 5.7382) construction
  line L4643 (37.737, 5.7382) -> (37.5369, 5.9382) construction
  line L4644 (37.5369, 5.9382) -> (37.29, 5.9382) construction
  spline S1473 degree 3 poles (37.29, 5.9382) (37.0431, 5.9382) (36.843, 5.7382) (36.843, 5.4914) knots 0 0 0 0 1 1 1 1
  line L4645 (37.29, 5.9382) -> (37.0431, 5.9382) construction
  line L4646 (37.0431, 5.9382) -> (36.843, 5.7382) construction
  line L4647 (36.843, 5.7382) -> (36.843, 5.4914) construction
  spline S1474 degree 3 poles (36.843, 5.4914) (36.843, 5.2446) (37.0431, 5.0443) (37.29, 5.0443) knots 0 0 0 0 1 1 1 1
  line L4648 (36.843, 5.4914) -> (36.843, 5.2446) construction
  line L4649 (36.843, 5.2446) -> (37.0431, 5.0443) construction
  line L4650 (37.0431, 5.0443) -> (37.29, 5.0443) construction
  spline S1475 degree 3 poles (37.29, 5.0443) (37.5369, 5.0443) (37.737, 5.2446) (37.737, 5.4914) knots 0 0 0 0 1 1 1 1
  line L4651 (37.29, 5.0443) -> (37.5369, 5.0443) construction
  line L4652 (37.5369, 5.0443) -> (37.737, 5.2446) construction
  line L4653 (37.737, 5.2446) -> (37.737, 5.4914) construction
  spline S1476 degree 3 poles (37.737, 0.3832) (37.737, 0.6299) (37.5369, 0.83) (37.29, 0.83) knots 0 0 0 0 1 1 1 1
  line L4654 (37.737, 0.3832) -> (37.737, 0.6299) construction
  line L4655 (37.737, 0.6299) -> (37.5369, 0.83) construction
  line L4656 (37.5369, 0.83) -> (37.29, 0.83) construction
  spline S1477 degree 3 poles (37.29, 0.83) (37.0431, 0.83) (36.843, 0.6299) (36.843, 0.3832) knots 0 0 0 0 1 1 1 1
  line L4657 (37.29, 0.83) -> (37.0431, 0.83) construction
  line L4658 (37.0431, 0.83) -> (36.843, 0.6299) construction
  line L4659 (36.843, 0.6299) -> (36.843, 0.3832) construction
  spline S1478 degree 3 poles (36.843, 0.3832) (36.843, 0.1364) (37.0431, -0.0639) (37.29, -0.0639) knots 0 0 0 0 1 1 1 1
  line L4660 (36.843, 0.3832) -> (36.843, 0.1364) construction
  line L4661 (36.843, 0.1364) -> (37.0431, -0.0639) construction
  line L4662 (37.0431, -0.0639) -> (37.29, -0.0639) construction
  spline S1479 degree 3 poles (37.29, -0.0639) (37.5369, -0.0639) (37.737, 0.1364) (37.737, 0.3832) knots 0 0 0 0 1 1 1 1
  line L4663 (37.29, -0.0639) -> (37.5369, -0.0639) construction
  line L4664 (37.5369, -0.0639) -> (37.737, 0.1364) construction
  line L4665 (37.737, 0.1364) -> (37.737, 0.3832) construction
  spline S1480 degree 3 poles (40.2911, 0.3832) (40.2911, 0.6299) (40.091, 0.83) (39.8441, 0.83) knots 0 0 0 0 1 1 1 1
  line L4666 (40.2911, 0.3832) -> (40.2911, 0.6299) construction
  line L4667 (40.2911, 0.6299) -> (40.091, 0.83) construction
  line L4668 (40.091, 0.83) -> (39.8441, 0.83) construction
  spline S1481 degree 3 poles (39.8441, 0.83) (39.5972, 0.83) (39.3971, 0.6299) (39.3971, 0.3832) knots 0 0 0 0 1 1 1 1
  line L4669 (39.8441, 0.83) -> (39.5972, 0.83) construction
  line L4670 (39.5972, 0.83) -> (39.3971, 0.6299) construction
  line L4671 (39.3971, 0.6299) -> (39.3971, 0.3832) construction
  spline S1482 degree 3 poles (39.3971, 0.3832) (39.3971, 0.1364) (39.5972, -0.0639) (39.8441, -0.0639) knots 0 0 0 0 1 1 1 1
  line L4672 (39.3971, 0.3832) -> (39.3971, 0.1364) construction
  line L4673 (39.3971, 0.1364) -> (39.5972, -0.0639) construction
  line L4674 (39.5972, -0.0639) -> (39.8441, -0.0639) construction
  spline S1483 degree 3 poles (39.8441, -0.0639) (40.091, -0.0639) (40.2911, 0.1364) (40.2911, 0.3832) knots 0 0 0 0 1 1 1 1
  line L4675 (39.8441, -0.0639) -> (40.091, -0.0639) construction
  line L4676 (40.091, -0.0639) -> (40.2911, 0.1364) construction
  line L4677 (40.2911, 0.1364) -> (40.2911, 0.3832) construction
  spline S1484 degree 3 poles (37.737, 2.9373) (37.737, 3.1841) (37.5369, 3.3841) (37.29, 3.3841) knots 0 0 0 0 1 1 1 1
  line L4678 (37.737, 2.9373) -> (37.737, 3.1841) construction
  line L4679 (37.737, 3.1841) -> (37.5369, 3.3841) construction
  line L4680 (37.5369, 3.3841) -> (37.29, 3.3841) construction
  spline S1485 degree 3 poles (37.29, 3.3841) (37.0431, 3.3841) (36.843, 3.1841) (36.843, 2.9373) knots 0 0 0 0 1 1 1 1
  line L4681 (37.29, 3.3841) -> (37.0431, 3.3841) construction
  line L4682 (37.0431, 3.3841) -> (36.843, 3.1841) construction
  line L4683 (36.843, 3.1841) -> (36.843, 2.9373) construction
  spline S1486 degree 3 poles (36.843, 2.9373) (36.843, 2.6905) (37.0431, 2.4902) (37.29, 2.4902) knots 0 0 0 0 1 1 1 1
  line L4684 (36.843, 2.9373) -> (36.843, 2.6905) construction
  line L4685 (36.843, 2.6905) -> (37.0431, 2.4902) construction
  line L4686 (37.0431, 2.4902) -> (37.29, 2.4902) construction
  spline S1487 degree 3 poles (37.29, 2.4902) (37.5369, 2.4902) (37.737, 2.6905) (37.737, 2.9373) knots 0 0 0 0 1 1 1 1
  line L4687 (37.29, 2.4902) -> (37.5369, 2.4902) construction
  line L4688 (37.5369, 2.4902) -> (37.737, 2.6905) construction
  line L4689 (37.737, 2.6905) -> (37.737, 2.9373) construction
  spline S1488 degree 3 poles (35.1829, 8.0455) (35.1829, 8.2923) (34.9826, 8.4923) (34.7358, 8.4923) knots 0 0 0 0 1 1 1 1
  line L4690 (35.1829, 8.0455) -> (35.1829, 8.2923) construction
  line L4691 (35.1829, 8.2923) -> (34.9826, 8.4923) construction
  line L4692 (34.9826, 8.4923) -> (34.7358, 8.4923) construction
  spline S1489 degree 3 poles (34.7358, 8.4923) (34.4891, 8.4923) (34.289, 8.2923) (34.289, 8.0455) knots 0 0 0 0 1 1 1 1
  line L4693 (34.7358, 8.4923) -> (34.4891, 8.4923) construction
  line L4694 (34.4891, 8.4923) -> (34.289, 8.2923) construction
  line L4695 (34.289, 8.2923) -> (34.289, 8.0455) construction
  spline S1490 degree 3 poles (34.289, 8.0455) (34.289, 7.7987) (34.4891, 7.5984) (34.7358, 7.5984) knots 0 0 0 0 1 1 1 1
  line L4696 (34.289, 8.0455) -> (34.289, 7.7987) construction
  line L4697 (34.289, 7.7987) -> (34.4891, 7.5984) construction
  line L4698 (34.4891, 7.5984) -> (34.7358, 7.5984) construction
  spline S1491 degree 3 poles (34.7358, 7.5984) (34.9826, 7.5984) (35.1829, 7.7987) (35.1829, 8.0455) knots 0 0 0 0 1 1 1 1
  line L4699 (34.7358, 7.5984) -> (34.9826, 7.5984) construction
  line L4700 (34.9826, 7.5984) -> (35.1829, 7.7987) construction
  line L4701 (35.1829, 7.7987) -> (35.1829, 8.0455) construction
  spline S1492 degree 3 poles (37.737, 8.0455) (37.737, 8.2923) (37.5369, 8.4923) (37.29, 8.4923) knots 0 0 0 0 1 1 1 1
  line L4702 (37.737, 8.0455) -> (37.737, 8.2923) construction
  line L4703 (37.737, 8.2923) -> (37.5369, 8.4923) construction
  line L4704 (37.5369, 8.4923) -> (37.29, 8.4923) construction
  spline S1493 degree 3 poles (37.29, 8.4923) (37.0431, 8.4923) (36.843, 8.2923) (36.843, 8.0455) knots 0 0 0 0 1 1 1 1
  line L4705 (37.29, 8.4923) -> (37.0431, 8.4923) construction
  line L4706 (37.0431, 8.4923) -> (36.843, 8.2923) construction
  line L4707 (36.843, 8.2923) -> (36.843, 8.0455) construction
  spline S1494 degree 3 poles (36.843, 8.0455) (36.843, 7.7987) (37.0431, 7.5984) (37.29, 7.5984) knots 0 0 0 0 1 1 1 1
  line L4708 (36.843, 8.0455) -> (36.843, 7.7987) construction
  line L4709 (36.843, 7.7987) -> (37.0431, 7.5984) construction
  line L4710 (37.0431, 7.5984) -> (37.29, 7.5984) construction
  spline S1495 degree 3 poles (37.29, 7.5984) (37.5369, 7.5984) (37.737, 7.7987) (37.737, 8.0455) knots 0 0 0 0 1 1 1 1
  line L4711 (37.29, 7.5984) -> (37.5369, 7.5984) construction
  line L4712 (37.5369, 7.5984) -> (37.737, 7.7987) construction
  line L4713 (37.737, 7.7987) -> (37.737, 8.0455) construction
  spline S1496 degree 3 poles (35.1829, 10.5996) (35.1829, 10.8464) (34.9826, 11.0465) (34.7358, 11.0465) knots 0 0 0 0 1 1 1 1
  line L4714 (35.1829, 10.5996) -> (35.1829, 10.8464) construction
  line L4715 (35.1829, 10.8464) -> (34.9826, 11.0465) construction
  line L4716 (34.9826, 11.0465) -> (34.7358, 11.0465) construction
  spline S1497 degree 3 poles (34.7358, 11.0465) (34.4891, 11.0465) (34.289, 10.8464) (34.289, 10.5996) knots 0 0 0 0 1 1 1 1
  line L4717 (34.7358, 11.0465) -> (34.4891, 11.0465) construction
  line L4718 (34.4891, 11.0465) -> (34.289, 10.8464) construction
  line L4719 (34.289, 10.8464) -> (34.289, 10.5996) construction
  spline S1498 degree 3 poles (34.289, 10.5996) (34.289, 10.3528) (34.4891, 10.1525) (34.7358, 10.1525) knots 0 0 0 0 1 1 1 1
  line L4720 (34.289, 10.5996) -> (34.289, 10.3528) construction
  line L4721 (34.289, 10.3528) -> (34.4891, 10.1525) construction
  line L4722 (34.4891, 10.1525) -> (34.7358, 10.1525) construction
  spline S1499 degree 3 poles (34.7358, 10.1525) (34.9826, 10.1525) (35.1829, 10.3528) (35.1829, 10.5996) knots 0 0 0 0 1 1 1 1
  line L4723 (34.7358, 10.1525) -> (34.9826, 10.1525) construction
  line L4724 (34.9826, 10.1525) -> (35.1829, 10.3528) construction
  line L4725 (35.1829, 10.3528) -> (35.1829, 10.5996) construction
  spline S1500 degree 3 poles (37.737, 10.5996) (37.737, 10.8464) (37.5369, 11.0465) (37.29, 11.0465) knots 0 0 0 0 1 1 1 1
  line L4726 (37.737, 10.5996) -> (37.737, 10.8464) construction
  line L4727 (37.737, 10.8464) -> (37.5369, 11.0465) construction
  line L4728 (37.5369, 11.0465) -> (37.29, 11.0465) construction
  spline S1501 degree 3 poles (37.29, 11.0465) (37.0431, 11.0465) (36.843, 10.8464) (36.843, 10.5996) knots 0 0 0 0 1 1 1 1
  line L4729 (37.29, 11.0465) -> (37.0431, 11.0465) construction
  line L4730 (37.0431, 11.0465) -> (36.843, 10.8464) construction
  line L4731 (36.843, 10.8464) -> (36.843, 10.5996) construction
  spline S1502 degree 3 poles (36.843, 10.5996) (36.843, 10.3528) (37.0431, 10.1525) (37.29, 10.1525) knots 0 0 0 0 1 1 1 1
  line L4732 (36.843, 10.5996) -> (36.843, 10.3528) construction
  line L4733 (36.843, 10.3528) -> (37.0431, 10.1525) construction
  line L4734 (37.0431, 10.1525) -> (37.29, 10.1525) construction
  spline S1503 degree 3 poles (37.29, 10.1525) (37.5369, 10.1525) (37.737, 10.3528) (37.737, 10.5996) knots 0 0 0 0 1 1 1 1
  line L4735 (37.29, 10.1525) -> (37.5369, 10.1525) construction
  line L4736 (37.5369, 10.1525) -> (37.737, 10.3528) construction
  line L4737 (37.737, 10.3528) -> (37.737, 10.5996) construction
  spline S1504 degree 3 poles (35.1829, 13.1537) (35.1829, 13.4005) (34.9826, 13.6006) (34.7358, 13.6006) knots 0 0 0 0 1 1 1 1
  line L4738 (35.1829, 13.1537) -> (35.1829, 13.4005) construction
  line L4739 (35.1829, 13.4005) -> (34.9826, 13.6006) construction
  line L4740 (34.9826, 13.6006) -> (34.7358, 13.6006) construction
  spline S1505 degree 3 poles (34.7358, 13.6006) (34.4891, 13.6006) (34.289, 13.4005) (34.289, 13.1537) knots 0 0 0 0 1 1 1 1
  line L4741 (34.7358, 13.6006) -> (34.4891, 13.6006) construction
  line L4742 (34.4891, 13.6006) -> (34.289, 13.4005) construction
  line L4743 (34.289, 13.4005) -> (34.289, 13.1537) construction
  spline S1506 degree 3 poles (34.289, 13.1537) (34.289, 12.9069) (34.4891, 12.7067) (34.7358, 12.7067) knots 0 0 0 0 1 1 1 1
  line L4744 (34.289, 13.1537) -> (34.289, 12.9069) construction
  line L4745 (34.289, 12.9069) -> (34.4891, 12.7067) construction
  line L4746 (34.4891, 12.7067) -> (34.7358, 12.7067) construction
  spline S1507 degree 3 poles (34.7358, 12.7067) (34.9826, 12.7067) (35.1829, 12.9069) (35.1829, 13.1537) knots 0 0 0 0 1 1 1 1
  line L4747 (34.7358, 12.7067) -> (34.9826, 12.7067) construction
  line L4748 (34.9826, 12.7067) -> (35.1829, 12.9069) construction
  line L4749 (35.1829, 12.9069) -> (35.1829, 13.1537) construction
  spline S1508 degree 3 poles (37.737, 13.1537) (37.737, 13.4005) (37.5369, 13.6006) (37.29, 13.6006) knots 0 0 0 0 1 1 1 1
  line L4750 (37.737, 13.1537) -> (37.737, 13.4005) construction
  line L4751 (37.737, 13.4005) -> (37.5369, 13.6006) construction
  line L4752 (37.5369, 13.6006) -> (37.29, 13.6006) construction
  spline S1509 degree 3 poles (37.29, 13.6006) (37.0431, 13.6006) (36.843, 13.4005) (36.843, 13.1537) knots 0 0 0 0 1 1 1 1
  line L4753 (37.29, 13.6006) -> (37.0431, 13.6006) construction
  line L4754 (37.0431, 13.6006) -> (36.843, 13.4005) construction
  line L4755 (36.843, 13.4005) -> (36.843, 13.1537) construction
  spline S1510 degree 3 poles (36.843, 13.1537) (36.843, 12.9069) (37.0431, 12.7067) (37.29, 12.7067) knots 0 0 0 0 1 1 1 1
  line L4756 (36.843, 13.1537) -> (36.843, 12.9069) construction
  line L4757 (36.843, 12.9069) -> (37.0431, 12.7067) construction
  line L4758 (37.0431, 12.7067) -> (37.29, 12.7067) construction
  spline S1511 degree 3 poles (37.29, 12.7067) (37.5369, 12.7067) (37.737, 12.9069) (37.737, 13.1537) knots 0 0 0 0 1 1 1 1
  line L4759 (37.29, 12.7067) -> (37.5369, 12.7067) construction
  line L4760 (37.5369, 12.7067) -> (37.737, 12.9069) construction
  line L4761 (37.737, 12.9069) -> (37.737, 13.1537) construction
  spline S1512 degree 3 poles (35.1829, 15.7078) (35.1829, 15.9546) (34.9826, 16.1547) (34.7358, 16.1547) knots 0 0 0 0 1 1 1 1
  line L4762 (35.1829, 15.7078) -> (35.1829, 15.9546) construction
  line L4763 (35.1829, 15.9546) -> (34.9826, 16.1547) construction
  line L4764 (34.9826, 16.1547) -> (34.7358, 16.1547) construction
  spline S1513 degree 3 poles (34.7358, 16.1547) (34.4891, 16.1547) (34.289, 15.9546) (34.289, 15.7078) knots 0 0 0 0 1 1 1 1
  line L4765 (34.7358, 16.1547) -> (34.4891, 16.1547) construction
  line L4766 (34.4891, 16.1547) -> (34.289, 15.9546) construction
  line L4767 (34.289, 15.9546) -> (34.289, 15.7078) construction
  spline S1514 degree 3 poles (34.289, 15.7078) (34.289, 15.461) (34.4891, 15.2608) (34.7358, 15.2608) knots 0 0 0 0 1 1 1 1
  line L4768 (34.289, 15.7078) -> (34.289, 15.461) construction
  line L4769 (34.289, 15.461) -> (34.4891, 15.2608) construction
  line L4770 (34.4891, 15.2608) -> (34.7358, 15.2608) construction
  spline S1515 degree 3 poles (34.7358, 15.2608) (34.9826, 15.2608) (35.1829, 15.461) (35.1829, 15.7078) knots 0 0 0 0 1 1 1 1
  line L4771 (34.7358, 15.2608) -> (34.9826, 15.2608) construction
  line L4772 (34.9826, 15.2608) -> (35.1829, 15.461) construction
  line L4773 (35.1829, 15.461) -> (35.1829, 15.7078) construction
  spline S1516 degree 3 poles (37.737, 15.7078) (37.737, 15.9546) (37.5369, 16.1547) (37.29, 16.1547) knots 0 0 0 0 1 1 1 1
  line L4774 (37.737, 15.7078) -> (37.737, 15.9546) construction
  line L4775 (37.737, 15.9546) -> (37.5369, 16.1547) construction
  line L4776 (37.5369, 16.1547) -> (37.29, 16.1547) construction